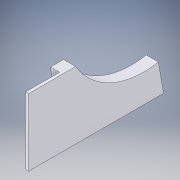
# Autodesk Inventor part: jam-protector
Saved by Autodesk Inventor 2019 (Build 230136000, 136)
## iProperties
Created: 2019-05-03
Part Number: jam-protector
Material: Generic
Document SubType Name: Modeling
Designer: Tesler
Density: 1 g/cm^3
Appearance: Default
Author: Tesler
Autodesk Inventor part; units mm, degrees
ref_plane "YZ Plane" through (0, 0, 0) normal (1, 0, 0) x (0, 1, 0)
ref_plane "XZ Plane" through (0, 0, 0) normal (0, 1, 0) x (-1, 0, 0)
ref_plane "XY Plane" through (0, 0, 0) normal (0, 0, 1) x (1, 0, 0)
sketch "Sketch1" plane through (0, 0, 0) normal (1, 0, 0) x (0, 1, 0)
  line L0 (0, 0) -> (0, -30.0167)
  line L1 (0, 0) -> (22.2363, 3.4344)
  line L2 (22.2363, 3.4344) -> (22.2363, -0.9099)
  arc A0 (22.2363, -0.9099) -> (9.8481, -28.2802) centre (35.4748, -23.3905) ccw
  line L3 (0, -30.0167) -> (9.8481, -28.2802)
  dimension "d27" = 30.0167
  dimension "d28" = 22.5
  dimension "d29" = 98.78
  dimension "d35" = 9.8481
  dimension "d36" = 80
  dimension "d37" = 26.089
  dimension "d38" = 13.2384
  constraints: 8 end point, 2 point on circle, 2 vertical, 1 centre point
  measures "d27" distance of L0.start L0.end
  measures "d28" distance of L0.start L1.end
  measures "d29" angle of L0 L1
  measures "d35" horizontal distance of L0.end L3.end
  measures "d36" angle of L0 L3
  measures "d37" radius of A0
  measures "d38" distance from line of L2 A0.centre
extrude "Extrusion1" add sketch "Sketch1" along normal blind 3
fillet "Fillet2" radius 2 1 edges at (1.5, 0, 0)
sketch "Sketch3" plane through (3, 0, 0) normal (1, 0, 0) x (0, 0, -1)
  line L0 (-3.4344, 22.2363) -> (-0.2618, 1.6947) projected
  line L1 (-3.4344, 22.2363) -> (-14.6844, 22.2363)
  line L2 (-14.6844, 22.2363) -> (-14.6844, 0)
  line L3 (1.7148, 0) -> (30.0167, 0) projected
  line L4 (-14.6844, 0) -> (30.0167, 0)
  arc A0 (0.9099, 22.2363) -> (28.2802, 9.8481) centre (23.3905, 35.4748) ccw projected
  line L5 (-3.4344, 22.2363) -> (0.9099, 22.2363)
  arc A1 (0.9099, 22.2363) -> (28.2802, 9.8481) centre (23.3905, 35.4748) ccw
  line L6 (30.0167, 0) -> (28.2802, 9.8481) projected
  line L7 (28.2802, 9.8481) -> (30.0167, 0)
  point P0 (0, 0)
  dimension "d32" = 11.25
  constraints: 10 end point, 2 collinear, 2 horizontal, 2 point on circle, 1 centre point, 1 concentric, 1 perpendicular
  measures "d32" distance of L0.start L1.end
extrude "Extrusion3" add sketch "Sketch3" along normal blind 1
body "Solid1"
